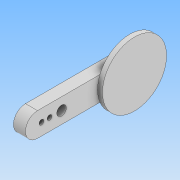
# Autodesk Inventor part: 震動臂
Saved by Autodesk Inventor 2021 (Build 250183000, 183)
## iProperties
Created: 2025-12-12
Part Number: 震動臂
Material: 一般
Document SubType Name: Modeling
Designer: User
Density: 1 g/cm^3
Appearance: 預設
Author: User
Autodesk Inventor part; units mm, degrees
ref_plane "YZ Plane" through (0, 0, 0) normal (1, 0, 0) x (0, 1, 0)
ref_plane "XZ Plane" through (0, 0, 0) normal (0, 1, 0) x (-1, 0, 0)
ref_plane "XY Plane" through (0, 0, 0) normal (0, 0, 1) x (1, 0, 0)
sketch "草圖1" plane through (0, 0, 0) normal (1, 0, 0) x (0, 1, 0)
  line L0 (75, 0) -> (-75, 0)
  line L1 (-75, 0) -> (-75, -300)
  line L2 (-75, -300) -> (75, -300)
  line L3 (75, -300) -> (75, 0)
  circle A0 centre (0, -100) radius 15
  circle A1 centre (0, -150) radius 15
  circle A2 centre (0, -225) radius 30
  line L4 (75, -300) -> (-75, -300)
  line L5 (-75, -300) -> (-75, -725)
  line L6 (-75, -725) -> (75, -725)
  line L7 (75, -725) -> (75, -300)
  point P0 (0, 0)
  point P1 (0, 0)
  dimension "d0" = 150
  dimension "d1" = 300
  dimension "d2" = 200
  dimension "d3" = 50
  dimension "d4" = 75
  dimension "d5" = 60
  dimension "d6" = 30
  dimension "d7" = 500
  constraints: 16 end point, 4 parallel, 3 centre point, 3 vertical alignment, 2 horizontal, 2 perpendicular, 1 coincident, 1 equal radius, 1 midpoint, 1 point on line
  measures "d0" distance of L0.start L0.end
  measures "d1" distance of L0.end L1.end
  measures "d2" distance from line of L2 A0.centre
  measures "d3" distance of A1.centre A0.centre
  measures "d4" distance of A2.centre A1.centre
  measures "d5" diameter of A2
  measures "d6" diameter of A1
  measures "d7" distance from line of A2.centre L6
extrude "擠出1" add sketch "草圖1" along normal mid plane 75
full round fillet "圓角1" first side at (-12.5, -75, -241.6667) centre faces at (12.5, -25, -725) second side at (-12.5, 75, -483.3333)
sketch "草圖2" plane through (37.5, 0, 0) normal (1, 0, 0) x (0, 0, -1)
  arc A0 (650, -75) -> (650, 75) centre (650, 0) ccw projected
  line L0 (650, 75) -> (0, 75) projected
  line L1 (0, 75) -> (0, -75) projected
  line L2 (0, -75) -> (650, -75) projected
  circle A1 centre (225, 0) radius 30 projected
  circle A2 centre (150, 0) radius 15 projected
  circle A3 centre (100, 0) radius 15 projected
  circle A4 centre (650, 0) radius 200
  point P0 (0, 0)
  dimension "d10" = 400
  constraints: 1 centre point, 1 coincident
  measures "d10" diameter of A4
extrude "擠出2" add sketch "草圖2" along normal blind 30 contours L2 A4 L0 A0 | A0 L0 A4 L2
fillet "圓角2" radius 75 2 edges at (0, 75, 0) (0, -75, 0)
